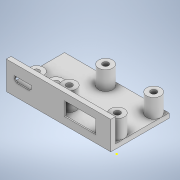
# Autodesk Inventor part: USB
Saved by Autodesk Inventor 2022 (Build 260153000, 153)
## iProperties
Created: 2021-07-07
Part Number: USB
Material: Generic
Document SubType Name: Modeling
Designer: anton
Density: 1 g/cm^3
Appearance: Default
Author: anton
Autodesk Inventor part; units mm, degrees
ref_plane "YZ Plane" through (0, 0, 0) normal (1, 0, 0) x (0, 1, 0)
ref_plane "XZ Plane" through (0, 0, 0) normal (0, 1, 0) x (-1, 0, 0)
ref_plane "XY Plane" through (0, 0, 0) normal (0, 0, 1) x (1, 0, 0)
sketch "Sketch1" plane through (0, 0, 0) normal (0, 1, 0) x (-1, 0, 0)
  line L0 (0, 0) -> (30, 0)
  line L1 (30, 0) -> (30, -25)
  line L2 (30, -25) -> (0, -25)
  line L3 (0, -25) -> (0, 0)
  dimension "d0" = 30
  dimension "d1" = 25
  constraints: 8 end point, 2 parallel, 1 horizontal, 1 perpendicular
  measures "d0" distance between parallel lines of L3 L1
  measures "d1" distance between parallel lines of L2 L0
extrude "Extrusion1" add sketch "Sketch1" along normal blind 2
sketch "Sketch2" plane through (0, 2, 0) normal (0, 1, 0) x (1, 0, 0)
  circle A0 centre (-5, 6) radius 3
  circle A1 centre (-5, 21.5) radius 3
  circle A2 centre (-25.5, 6) radius 3
  circle A3 centre (-25.5, 21.5) radius 3
  line L0 (0, 0) -> (0, 25) projected
  line L1 (0, 25) -> (-30, 25) projected
  dimension "d4" = 15.5
  dimension "d5" = 15.5
  dimension "d6" = 20.5
  dimension "d7" = 20.5
  dimension "d8" = 0
  dimension "d9" = 0
  dimension "d10" = 6
  dimension "d11" = 6
  dimension "d12" = 6
  dimension "d13" = 6
  dimension "d14" = 5
  dimension "d15" = 3.5
  constraints: 4 centre point
  measures "d4" distance of A3.centre A2.centre
  measures "d5" distance of A1.centre A0.centre
  measures "d6" distance of A0.centre A2.centre
  measures "d7" distance of A1.centre A3.centre
  measures "d8" horizontal distance of A0.centre A1.centre
  measures "d9" vertical distance of A1.centre A3.centre
  measures "d10" diameter of A2
  measures "d11" diameter of A3
  measures "d12" diameter of A1
  measures "d13" diameter of A0
  measures "d14" distance from line of L0 A1.centre
  measures "d15" distance from line of L1 A3.centre
extrude "Extrusion2" add sketch "Sketch2" along normal blind 8
sketch "Sketch3" plane through (-25.5, 10, -6) normal (0, 1, 0) x (1, 0, 0)
  circle A0 centre (20.5, 0) radius 3 projected
  circle A1 centre (20.5, 0) radius 1.25
  circle A2 centre (20.5, 15.5) radius 3 projected
  circle A3 centre (20.5, 15.5) radius 1.25
  circle A4 centre (0, 15.5) radius 3 projected
  circle A5 centre (0, 15.5) radius 1.25
  circle A6 centre (0, 0) radius 3 projected
  circle A7 centre (0, 0) radius 1.25
  point P0 (25.5, -6)
  dimension "d18" = 2.5
  dimension "d19" = 2.5
  dimension "d20" = 2.5
  dimension "d21" = 2.5
  constraints: 4 centre point, 4 coincident
  measures "d18" diameter of A7
  measures "d19" diameter of A5
  measures "d20" diameter of A3
  measures "d21" diameter of A1
extrude "Extrusion3" cut sketch "Sketch3" against normal blind 4 contours A1 | A3 | A5 | A7
sketch "Sketch4" plane through (0, 2, 0) normal (0, 1, 0) x (1, 0, 0)
  line L0 (-30, 25) -> (-30, 0) projected
  line L1 (0, 0) -> (0, 25) projected
  line L2 (-30, 0.2) -> (0, 0.2)
  line L3 (0, 0.2) -> (0, 2.2)
  line L4 (0, 2.2) -> (-30, 2.2)
  line L5 (-30, 2.2) -> (-30, 0.2)
  circle A0 centre (-25.5, 6) radius 1.25 projected
  point P0 (0, 0.2)
  dimension "d28" = 5.8
  dimension "d29" = 2
  constraints: 8 end point, 2 parallel, 2 point on line, 1 horizontal, 1 perpendicular
  measures "d28" distance from line of L2 A0.centre
  measures "d29" distance between parallel lines of L2 L4
extrude "Extrusion4" add sketch "Sketch4" along normal blind 10 contours L4 L1 L2 L0
sketch "Sketch5" plane through (-30, 2, -0.2) normal (0, 0, 1) x (1, 0, 0)
  line L0 (21.7, 7) -> (8.3, 7)
  line L1 (8.3, 7) -> (8.3, 1.2)
  line L2 (8.3, 1.2) -> (21.7, 1.2)
  line L3 (21.7, 1.2) -> (21.7, 7)
  line L4 (28, 8) -> (22, 8) projected
  line L5 (0, 0) -> (0, 10) projected
  point P0 (30, -2)
  point P1 (25, 8)
  dimension "d32" = 13.4
  dimension "d33" = 5.8
  dimension "d36" = 1
  dimension "d37" = 8.3
  constraints: 8 end point, 2 parallel, 1 horizontal, 1 perpendicular
  measures "d32" distance between parallel lines of L3 L1
  measures "d33" distance between parallel lines of L2 L0
  measures "d36" distance between parallel lines of L4 L0
  measures "d37" distance between parallel lines of L5 L1
extrude "Extrusion5" cut sketch "Sketch5" against normal blind 10
sketch "Sketch6" plane through (0, 2, 0) normal (0, 1, 0) x (1, 0, 0)
  line L0 (0, 25) -> (-30, 25) projected
  line L1 (-30, 0.2) -> (0, 0.2) projected
  line L2 (-29.3171, 25) -> (-1.9814, 25)
  line L3 (-1.9814, 25) -> (-1.9814, 0.2)
  line L4 (-1.9814, 0.2) -> (-29.3171, 0.2)
  line L5 (-29.3171, 0.2) -> (-29.3171, 25)
  line L6 (-32.5014, 28.1843) -> (1.2029, 28.1843)
  line L7 (1.2029, 28.1843) -> (1.2029, -2.9843)
  line L8 (1.2029, -2.9843) -> (-32.5014, -2.9843)
  line L9 (-32.5014, -2.9843) -> (-32.5014, 28.1843)
  point P0 (-29.3171, 0.2)
  constraints: 16 end point, 4 parallel, 2 perpendicular, 2 point on line, 1 horizontal, 3 other
extrude "Extrusion6" cut sketch "Sketch6" along normal mid plane 100
sketch "Sketch7" plane through (-1.9814, 2, -2.2) normal (0, 0, -1) x (-1, 0, 0)
  line L0 (0, 0) -> (27.3358, 0) projected
  line L1 (5.0186, 8.5) -> (21.0186, 8.5)
  line L2 (21.0186, 8.5) -> (21.0186, 0)
  line L3 (21.0186, 0) -> (5.0186, 0)
  line L4 (5.0186, 0) -> (5.0186, 8.5)
  line L5 (6.3186, 1.2) -> (6.3186, 7) projected
  line L6 (6.3186, 7) -> (19.7186, 7) projected
  point P0 (-1.9814, -2)
  point P1 (5.0186, 0)
  dimension "d42" = 16
  dimension "d43" = 1.3
  dimension "d44" = 1.5
  constraints: 8 end point, 2 parallel, 1 horizontal, 1 perpendicular, 1 point on line
  measures "d42" distance between parallel lines of L2 L4
  measures "d43" distance between parallel lines of L5 L4
  measures "d44" distance between parallel lines of L6 L1
extrude "Extrusion7" cut sketch "Sketch7" against normal blind 1.5
sketch "Sketch12" plane through (0, 2, 0) normal (0, 1, 0) x (1, 0, 0)
  line L0 (-29.3171, 0.2) -> (-1.9814, 0.2) projected
  line L1 (-29.3171, 0.2) -> (-46.5, 0.2)
  line L2 (-46.5, 0.2) -> (-46.5, 25)
  line L3 (-46.5, 25) -> (-29.3171, 25)
  line L4 (-29.3171, 25) -> (-29.3171, 0.2)
  circle A0 centre (-25.5, 6) radius 3 projected
  point P0 (0, 0)
  dimension "d49" = 18
  constraints: 8 end point, 2 parallel, 1 horizontal, 1 perpendicular
  measures "d49" distance edge to line of A0 L2
extrude "Extrusion8" add sketch "Sketch12" against normal blind 2 contours L1 L2 L3 L4
sketch "Sketch13" plane through (0, 2, 0) normal (0, 1, 0) x (1, 0, 0)
  line L0 (-29.3171, 2.2) -> (-23, 2.2) projected
  line L1 (-46.5, 25) -> (-46.5, 0.2) projected
  line L2 (-29.3171, 2.2) -> (-46.5, 2.2)
  line L3 (-46.5, 2.2) -> (-46.5, 0.2)
  line L4 (-46.5, 0.2) -> (-29.3171, 0.2)
  line L5 (-29.3171, 0.2) -> (-29.3171, 2.2)
  point P0 (0, 0)
  constraints: 8 end point, 2 parallel, 1 horizontal, 1 perpendicular
extrude "Extrusion9" add sketch "Sketch13" along normal up to surface (10 mm away)
sketch "Sketch14" plane through (0, 2, 0) normal (0, 1, 0) x (1, 0, 0)
  line L0 (-46.5, 0.2) -> (-46.5, 25) projected
  line L1 (-1.9814, 0.2) -> (-46.5, 0.2) projected
  line L2 (-46.5, 25) -> (-32.5, 25)
  line L3 (-32.5, 25) -> (-32.5, 0.2)
  line L4 (-32.5, 0.2) -> (-46.5, 0.2)
  line L5 (-46.5, 0.2) -> (-46.5, 25)
  circle A0 centre (-35.35, 10.2) radius 3
  arc A1 (-46.5, 9.2633) -> (-46.5, 11.1367) centre (-43.65, 10.2) ccw
  point P0 (0, 0)
  point P1 (-32.5, 9.2633)
  point P2 (-32.5, 11.1367)
  dimension "d54" = 14
  dimension "d55" = 10
  dimension "d56" = 10
  dimension "d57" = 8.3
  dimension "d58" = 6
  dimension "d59" = 6
  dimension "d60" = 2.85
  constraints: 8 end point, 3 point on line, 2 centre point, 2 parallel, 2 point on circle, 1 horizontal, 1 perpendicular
  measures "d54" distance between parallel lines of L0 L3
  measures "d55" distance from line of L1 A0.centre
  measures "d56" distance from line of L1 A1.centre
  measures "d57" distance of A1.centre A0.centre
  measures "d58" diameter of A0
  measures "d59" diameter of A1
  measures "d60" distance from line of L3 A0.centre
extrude "Extrusion10" add sketch "Sketch14" along normal blind 1.9 contours L0 A1 | A0 L3 picked at (-36.2658, 10.5122)
sketch "Sketch15" plane through (0, 3.9, 0) normal (0, 1, 0) x (1, 0, 0)
  arc A0 (-32.5, 11.1367) -> (-32.5, 9.2633) centre (-35.35, 10.2) ccw projected
  circle A1 centre (-35.35, 10.2) radius 1.25
  arc A2 (-46.5, 9.2633) -> (-46.5, 11.1367) centre (-43.65, 10.2) ccw projected
  circle A3 centre (-43.65, 10.2) radius 1.25
  point P0 (0, 0)
  dimension "d63" = 2.5
  dimension "d64" = 2.5
  constraints: 2 centre point, 2 coincident
  measures "d63" diameter of A1
  measures "d64" diameter of A3
extrude "Extrusion11" cut sketch "Sketch15" against normal blind 4
sketch "Sketch16" plane through (-1.9814, 2, -2.2) normal (0, 0, -1) x (-1, 0, 0)
  line L0 (33.7186, 5.6) -> (41.1186, 5.6)
  line L1 (41.1186, 5.6) -> (41.1186, 4.3)
  line L2 (40.1186, 3.3) -> (34.7186, 3.3)
  line L3 (33.7186, 4.3) -> (33.7186, 5.6)
  line L4 (36.3686, 0) -> (36.3686, 1.9) projected
  line L5 (36.3686, 1.5842) -> (36.3686, 2.8612)
  line L6 (38.6686, 0) -> (38.6686, 1.9) projected
  line L7 (38.6686, 1.3572) -> (38.6686, 2.8612)
  line L8 (36.3686, 1.9) -> (30.5186, 1.9) projected
  line L9 (34.7186, 3.3) -> (40.1186, 3.3)
  line L10 (34.7186, 3.3) -> (33.7186, 4.3)
  line L11 (40.1186, 3.3) -> (41.1186, 4.3)
  point P0 (-1.9814, -2)
  dimension "d68" = 7.4
  dimension "d69" = 2.3
  dimension "d70" = 2.65
  dimension "d71" = 1.4
  dimension "d75" = 1
  dimension "d76" = 1
  dimension "d77" = 135
  constraints: 18 end point, 2 collinear, 2 horizontal, 2 parallel, 2 perpendicular, 2 point on line
  measures "d68" distance between parallel lines of L1 L3
  measures "d69" distance between parallel lines of L2 L0
  measures "d70" distance between parallel lines of L3 L5
  measures "d71" distance between parallel lines of L8 L2
  measures "d75" horizontal distance of L3.start L2.end
  measures "d76" horizontal distance of L1.end L2.start
  measures "d77" angle of L2 L10
extrude "Extrusion12" cut sketch "Sketch16" against normal blind 4
sketch "Sketch17" plane through (-1.9814, 2, -2.2) normal (0, 0, -1) x (-1, 0, 0)
  line L0 (0, 0) -> (44.5186, 0) projected
  line L1 (29.5186, 3.5) -> (44.5186, 3.5)
  line L2 (44.5186, 3.5) -> (44.5186, 0)
  line L3 (44.5186, 0) -> (29.5186, 0)
  line L4 (29.5186, 0) -> (29.5186, 3.5)
  line L5 (36.3686, 1.9) -> (30.5186, 1.9) projected
  line L6 (36.3686, 1.9) -> (38.6686, 1.9)
  line L7 (38.6686, 0) -> (38.6686, 1.9) projected
  line L8 (37.5186, 1.9) -> (37.5186, 2.6823)
  line L9 (32.7186, 3.5) -> (42.1186, 3.5)
  line L10 (42.1186, 3.5) -> (42.1186, 6.6)
  line L11 (42.1186, 6.6) -> (32.7186, 6.6)
  line L12 (32.7186, 6.6) -> (32.7186, 3.5)
  line L13 (33.7186, 5.6) -> (41.1186, 5.6) projected
  line L14 (33.7186, 4.3) -> (33.7186, 5.6) projected
  line L15 (41.1186, 5.6) -> (41.1186, 4.3) projected
  point P0 (-1.9814, -2)
  point P1 (29.5186, 0)
  dimension "d80" = 1.6
  dimension "d81" = 8
  dimension "d82" = 1
  dimension "d83" = 1
  dimension "d84" = 1
  constraints: 20 end point, 4 parallel, 3 horizontal, 2 perpendicular, 2 point on line, 1 midpoint, 1 vertical
  measures "d80" distance between parallel lines of L5 L1
  measures "d81" distance between parallel lines of L4 L8
  measures "d82" distance between parallel lines of L13 L11
  measures "d83" distance between parallel lines of L14 L12
  measures "d84" distance between parallel lines of L15 L10
extrude "Extrusion13" cut sketch "Sketch17" against normal blind 1.5
sketch "Sketch18" plane through (-1.9814, 2, -0.7) normal (0, 0, -1) x (-1, 0, 0)
  point P0 (-1.9814, -2)
body "Solid1"
